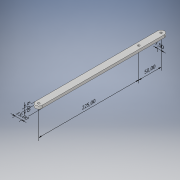
# Autodesk Inventor part: GraspArm
Saved by Autodesk Inventor 2019 (Build 230136000, 136)
## iProperties
Created: 2018-06-10
Part Number: GraspArm
Material: Ogólny
Document SubType Name: Modeling
Designer: Kamil
Density: 1 g/cm^3
Appearance: Domyślna
Author: Kamil
## iProperties of the stored document GraspArm_Drukowanie 3D.ipt
Created: 2018-06-10
Part Number: GraspArm_Drukowanie 3D
Material: Ogólny
Document SubType Name: Modeling
Designer: Kamil
Density: 1 g/cm^3
Appearance: Domyślna
Author: Kamil
Autodesk Inventor part; units mm, degrees
ref_plane "YZ Plane" through (0, 0, 0) normal (1, 0, 0) x (0, 1, 0)
ref_plane "XZ Plane" through (0, 0, 0) normal (0, 1, 0) x (-1, 0, 0)
ref_plane "XY Plane" through (0, 0, 0) normal (0, 0, 1) x (1, 0, 0)
sketch "Szkic3" plane through (0, 0, 0) normal (0, 1, 0) x (-1, 0, 0)
  line L0 (0, -145) -> (0, -145)
  line L1 (7.5, -137.5) -> (7.5, 137.5)
  line L2 (0, 145) -> (0, 145)
  line L3 (-7.5, 137.5) -> (-7.5, -137.5)
  circle A0 centre (0, 137.5) radius 2.25
  circle A1 centre (0, -137.5) radius 2.25
  circle A2 centre (0, -87.5) radius 2.25
  arc A3 (7.5, 137.5) -> (0, 145) centre (0, 137.5) ccw
  arc A4 (0, 145) -> (-7.5, 137.5) centre (0, 137.5) ccw
  arc A5 (0, -145) -> (7.5, -137.5) centre (0, -137.5) ccw
  arc A6 (-7.5, -137.5) -> (0, -145) centre (0, -137.5) ccw
  point P0 (0, 0)
  point P1 (7.5, 145)
  point P2 (7.5, -145)
  point P3 (-7.5, 145)
  point P4 (0, 145)
  point P5 (7.1121, 137.5)
  point P6 (-7.1121, 137.5)
  point P7 (7.1121, -137.5)
  point P8 (0, -145)
  point P9 (-7.1121, -137.5)
  point P10 (0, 145)
  dimension "d11" = 15
  dimension "d12" = 290
  dimension "d13" = 4.5
  dimension "d14" = 4.5
  dimension "d15" = 4.5
  dimension "d16" = 7.5
  dimension "d17" = 7.5
  constraints: 8 end point, 8 point on circle, 8 point on line, 8 tangent, 7 centre point, 2 equal radius, 2 midpoint, 2 parallel, 1 coincident, 1 horizontal, 1 perpendicular
  measures "d11" distance of point (-7.5, 145) point (7.5, 145)
  measures "d12" distance of point (7.5, 145) point (7.5, -145)
  measures "d13" diameter of A0
  measures "d14" diameter of A1
  measures "d15" diameter of A2
  measures "d16" radius of A3
  measures "d17" radius of A4
extrude "Wyciągnięcie proste2" add sketch "Szkic3" along normal blind 6
